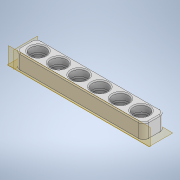
# Autodesk Inventor part: Test_Well6x1
Saved by Autodesk Inventor 2022 (Build 260153000, 153)
## iProperties
Created: 2021-11-23
Part Number: Test_Well6x1
Material: Generic
Document SubType Name: Modeling
Designer: Gareth
Density: 1 g/cm^3
Appearance: Default
Author: Gareth
Autodesk Inventor part; units mm, degrees
sketch "Sketch1" plane through (0, 0, 0) normal (0, 1, 0) x (-1, 0, 0)
  line L0 (0, 0) -> (-125, 0)
  line L1 (-125, 0) -> (-125, -21)
  line L2 (-125, -21) -> (0, -21)
  line L3 (0, -21) -> (0, 0)
  dimension "d0" = 125
  dimension "d1" = 21
  constraints: 8 end point, 2 parallel, 1 horizontal, 1 perpendicular
  measures "d0" distance of L1.end L2.end
  measures "d1" distance of L0.end L1.end
extrude "Extrusion1" add sketch "Sketch1" along normal blind 15
sketch "Sketch2" plane through (0, 15, 0) normal (0, 1, 0) x (1, 0, 0)
  line L0 (125, 21) -> (0, 21) projected
  line L1 (0, 21) -> (0, 0) projected
  line L2 (125, 0) -> (125, 21) projected
  line L3 (0, 0) -> (125, 0) projected
  circle A0 centre (12, 10.5) radius 7.5
  dimension "d4" = 15
  dimension "d5" = 10.5
  dimension "d6" = 12
  constraints: 1 centre point
  measures "d4" diameter of A0
  measures "d5" distance from line of L0 A0.centre
  measures "d6" distance from line of L1 A0.centre
extrude "Extrusion2" cut sketch "Sketch2" against normal blind 7.5 contours A0
fillet "Fillet1" radius 1 2 edges at (4.5, 7.5, -10.5) (4.5, 15, -10.5)
pattern_linear "Rectangular Pattern2" count 6 spacing 20 along (1, 0, 0) of "Extrusion2", "Fillet1"
fillet "Fillet2" radius 5 4 edges at (0, 7.5, 0) (125, 7.5, 0) (0, 7.5, -21) (125, 7.5, -21)
fillet "Fillet3" radius 1 16 edges at (62.5, 15, -21) (1.4645, 15, -19.5355) (0, 15, -10.5) (1.4645, 15, -1.4645) (62.5, 15, 0) (123.5355, 15, -1.4645) (125, 15, -10.5) (123.5355, 15, -19.5355) (1.4645, 0, -19.5355) (0, 0, -10.5) (1.4645, 0, -1.4645) (62.5, 0, 0) (123.5355, 0, -1.4645) (125, 0, -10.5) (123.5355, 0, -19.5355) (62.5, 0, -21)
body "Solid1"
